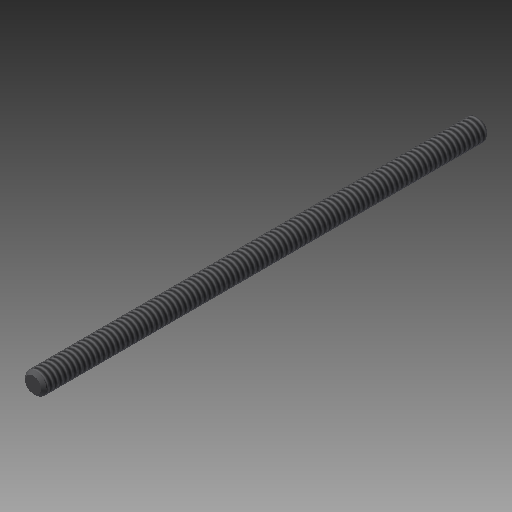
# Autodesk Inventor part: D-47932-SS-2.317
Saved by Autodesk Inventor 2017 (Build 210142000, 142)
## iProperties
Category: PARTsolutions
Company: BIMBA
Created: 2017-01-25
Part Number: D-47932-SS-2.317
Catalog Web Link: www.cadenas.de
Description: BIF Tie Rod-Bimba FLAT-1
Vendor: BIMBA
Document SubType Name: Modeling
Designer: psAdmin
Manufacturer: BIMBA
Mass: 0.372904 g
Surface Area: 5.34347 cm^2
Volume: 0.372904 cm^3
Density: 1 g/cm^3
Material: Generic
Appearance: PSOLRGB-192-192-192
PSOL_IDENT_0: {$CADENAS_DATA\23d-libs\bimba\bimba\bimba_imperial\bimba_full_line\flat_cylinders\fo1\bif_tie_rod.pr
PSOL_IDENT_1: j},180 {VTYP=3D},{NB=D-47932-SS-2.317},{LINA=D-47932-SS-2.317},{NN=BIF Tie Rod},{DATE=01.12.2016 06:
PSOL_IDENT_2: 16:11},{GEOMDATE=20.05.2016 08:43:22},{VERSION=},{LINEID=10},{LINESUBID=-1},{WBVAR=L}  {NB=D-47932-S
PSOL_IDENT_3: S-2.317},{LINA=D-47932-SS-2.317},{KT=DUMMY},{PN=D-47932-SS-2.317},{MODEL=D-47932-SS},{NDM=0.112},{L=
PSOL_IDENT_4: 2.31700},{HWL=0.070}
NN: BIF Tie Rod
NT: Bimba FLAT-1
NB: D-47932-SS-2.317
NBSYN: $PN.
LINA: D-47932-SS-2.317
PN: D-47932-SS-2.317
MODEL: D-47932-SS
NDM: 0.112
L: 2.31700
HWL: 0.070
SUPPLIER: BIMBA
ARTICLENO: D-47932-SS-2.317
BOMINFO: D-47932-SS-2.317
CREATOR: CADENAS GmbH
Title: D-47932-SS-2.317
Author: Cadenas PARTsolutions
Comments: Bimba FLAT-1
Autodesk Inventor part; units mm, degrees
sketch "Sketch_1" plane through (0, 0, 0) normal (1, 0, 0) x (0, 1, 0)
  line L0 (0, -57.0738) -> (0, 1.778)
  line L1 (0, 1.778) -> (1.0439, 1.778)
  line L2 (1.0439, 1.778) -> (1.4224, 1.3995)
  line L3 (1.4224, 1.3995) -> (1.4224, -56.6953)
  line L4 (1.4224, -56.6953) -> (1.0439, -57.0738)
  line L5 (1.0439, -57.0738) -> (0, -57.0738)
  line L6 (0, -57.0738) -> (0, 1.778)
  constraints: 14 end point
revolve "Revolution1" add sketch "Sketch_1" angle 360 about axis through (0, 0, -57.0738) along (0, 0, -1)
thread "Thread1" size "4-40 UNC" class "2A" standard "ANSI Unified Screw Threads" full length
ref_plane "screw_XY" through (0, 0, 0) normal (0, 0, 1) x (1, 0, 0)
ref_plane "screw_YZ" through (0, 0, 0) normal (1, 0, 0) x (0, 1, 0)
ref_plane "screw_ZX" through (0, 0, 0) normal (0, 1, 0) x (0, 0, 1)
body "Solid1"
